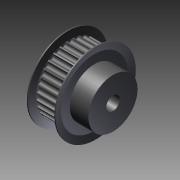
# Autodesk Inventor part: zrr_htd_3m9_6_17023200
Saved by Autodesk Inventor 2011 SP1 (Build 150282100, 282)
## iProperties
Created: 2018-07-07
Part Number: zrr_htd_3m9_6_17023200
Catalog Web Link: www.cadenas.de
Description: zrr_htd_3m9-HTD Pulleys Profile 3M, Timing Belt Width 9 mm
Vendor: MAEDLER
Document SubType Name: Modeling
Designer: psAdmin
Manufacturer: MAEDLER
Mass: 41 g
Surface Area: 52.9577 cm^2
Volume: 10.7438 cm^3
Density: 1 g/cm^3
Category: PARTsolutions
Company: MAEDLER
Title: zrr_htd_3m9_6_17023200
Author: Cadenas PARTsolutions
Comments: HTD Pulleys Profile 3M, Timing Belt Width 9 mm
PSOL_IDENT_0: {$CADENAS_DATA\23d-libs\maedler\antriebselemente\zahnriemenraeder_zahnriemen\zahnriemenraeder\htd-pr
PSOL_IDENT_1: ofil\zrr_htd_3m09.prj},194 {VTYP=3D},{NB=zrr_htd_3m9_6_17023200},{LINA=zrr_htd_3m9_6_17023200},{NN=z
PSOL_IDENT_2: rr_htd_3m9},{DATE=31.01.2018 13:45:46},{GEOMDATE=31.01.2018 13:45:46},{VERSION=},{LINEID=340},{LINES
PSOL_IDENT_3: UBID=-1},{WBVAR=BX}  {NB=zrr_htd_3m9_6_17023200},{LINA=zrr_htd_3m9_6_17023200},{KT=DUMMY},{ARTNR=170
PSOL_IDENT_4: 23200},{PDF=PDF Katalogseite},{AUSF=32-3M-09-1F},{MAT=Aluminium},{ZTL=3.000},{ZRB=9.000},{Z=32.000},
PSOL_IDENT_5: {AUS=1F},{ZS=29.800},{BS=36.000},{DO=30.560},{ND=22.000},{B=12.800},{L=20.600},{I=0.000},{VB=6.000},
PSOL_IDENT_6: {FB=13.500},{BX=6},{GEW=41.000},{ZT=1.200},{ZB=1.800},{T=1.000},{BB=1.000}
NN: zrr_htd_3m9
NT: HTD-Zahnriemenräder Profil 3M, Zahnriemenbreite 9mm
NB: zrr_htd_3m9_6_17023200
NBSYN: zrr_htd_3m9_$BX._$ARTNR.
LINA: zrr_htd_3m9_6_17023200
ARTNR: 17023200
PDF: PDF Katalogseite
AUSF: 32-3M-09-1F
MAT: Aluminium
ZTL: 3.000
ZRB: 9.000
Z: 32.000
AUS: 1F
ZS: 29.800
BS: 36.000
DO: 30.560
ND: 22.000
B: 12.800
L: 20.600
I: 0.000
VB: 6.000
FB: 13.500
BX: 6
GEW: 41.000
ZT: 1.200
ZB: 1.800
T: 1.000
BB: 1.000
SUPPLIER: MAEDLER
ARTICLENO: zrr_htd_3m9_6_17023200
BOMINFO: zrr_htd_3m9_6_17023200
CREATOR: CADENAS GmbH
Autodesk Inventor part; units mm, degrees
ref_plane "YZ Plane" through (0, 0, 0) normal (1, 0, 0) x (0, 1, 0)
ref_plane "XZ Plane" through (0, 0, 0) normal (0, 1, 0) x (-1, 0, 0)
ref_plane "XY Plane" through (0, 0, 0) normal (0, 0, 1) x (1, 0, 0)
sketch "Sketch_3" plane through (0, 0, 0) normal (0, 0, 1) x (1, 0, 0)
  line L0 (500, 0) -> (-500, 0)
  line L1 (0, 0) -> (0, 18)
  line L2 (0, 18) -> (0.4534, 18)
  line L3 (0.4534, 18) -> (1, 14.9)
  line L4 (1, 14.9) -> (11.8, 14.9)
  line L5 (11.8, 14.9) -> (12.3466, 18)
  line L6 (12.3466, 18) -> (12.8, 18)
  line L7 (12.8, 18) -> (12.2534, 14.9)
  line L8 (12.2534, 14.9) -> (12.2534, 11)
  line L9 (12.2534, 11) -> (20.6, 11)
  line L10 (20.6, 11) -> (20.6, 0)
  line L11 (20.6, 0) -> (0, 0)
  constraints: 24 end point
revolve "Revolution1" add sketch "Sketch_3" angle 360 about axis through (500, 0, 0) along (1, 0, 0)
sketch "Sketch_4" plane through (1, 0, 0) normal (1, 0, 0) x (0, 0, -1)
  circle A0 centre (0, 0) radius 206
  arc A1 (-14.8517, -1.199) -> (-14.8283, -1.4605) centre (0, 0) ccw
  arc A2 (-14.8283, -1.4605) -> (-14.8002, -1.7214) centre (0, 0) ccw
  arc A3 (-14.3324, -4.0734) -> (-14.8002, -1.7214) centre (-14.6137, -2.9068) ccw
  arc A4 (-14.3324, -4.0734) -> (-14.2584, -4.3252) centre (0, 0) ccw
  arc A5 (-14.2584, -4.3252) -> (-14.18, -4.5757) centre (0, 0) ccw
  arc A6 (-13.2623, -6.7912) -> (-14.18, -4.5757) centre (-13.7658, -5.702) ccw
  arc A7 (-13.2623, -6.7912) -> (-13.1406, -7.0238) centre (0, 0) ccw
  arc A8 (-13.1406, -7.0238) -> (-13.0149, -7.2542) centre (0, 0) ccw
  arc A9 (-11.6826, -9.2481) -> (-13.0149, -7.2542) centre (-12.3889, -8.278) ccw
  arc A10 (-11.6826, -9.2481) -> (-11.5179, -9.4525) centre (0, 0) ccw
  arc A11 (-11.5179, -9.4525) -> (-11.3496, -9.6539) centre (0, 0) ccw
  arc A12 (-9.6539, -11.3496) -> (-11.3496, -9.6539) centre (-10.5359, -10.5359) ccw
  arc A13 (-9.6539, -11.3496) -> (-9.4525, -11.5179) centre (0, 0) ccw
  arc A14 (-9.4525, -11.5179) -> (-9.2481, -11.6826) centre (0, 0) ccw
  arc A15 (-7.2542, -13.0149) -> (-9.2481, -11.6826) centre (-8.278, -12.3889) ccw
  arc A16 (-7.2542, -13.0149) -> (-7.0238, -13.1406) centre (0, 0) ccw
  arc A17 (-7.0238, -13.1406) -> (-6.7912, -13.2623) centre (0, 0) ccw
  arc A18 (-4.5757, -14.18) -> (-6.7912, -13.2623) centre (-5.702, -13.7658) ccw
  arc A19 (-4.5757, -14.18) -> (-4.3252, -14.2584) centre (0, 0) ccw
  arc A20 (-4.3252, -14.2584) -> (-4.0734, -14.3324) centre (0, 0) ccw
  arc A21 (-1.7214, -14.8002) -> (-4.0734, -14.3324) centre (-2.9068, -14.6137) ccw
  arc A22 (-1.7214, -14.8002) -> (-1.4605, -14.8283) centre (0, 0) ccw
  arc A23 (-1.4605, -14.8283) -> (-1.199, -14.8517) centre (0, 0) ccw
  arc A24 (1.199, -14.8517) -> (-1.199, -14.8517) centre (0, -14.9) ccw
  arc A25 (1.199, -14.8517) -> (1.4605, -14.8283) centre (0, 0) ccw
  arc A26 (1.4605, -14.8283) -> (1.7214, -14.8002) centre (0, 0) ccw
  arc A27 (4.0734, -14.3324) -> (1.7214, -14.8002) centre (2.9068, -14.6137) ccw
  arc A28 (4.0734, -14.3324) -> (4.3252, -14.2584) centre (0, 0) ccw
  arc A29 (4.3252, -14.2584) -> (4.5757, -14.18) centre (0, 0) ccw
  arc A30 (6.7912, -13.2623) -> (4.5757, -14.18) centre (5.702, -13.7658) ccw
  arc A31 (6.7912, -13.2623) -> (7.0238, -13.1406) centre (0, 0) ccw
  arc A32 (7.0238, -13.1406) -> (7.2542, -13.0149) centre (0, 0) ccw
  arc A33 (9.2481, -11.6826) -> (7.2542, -13.0149) centre (8.278, -12.3889) ccw
  arc A34 (9.2481, -11.6826) -> (9.4525, -11.5179) centre (0, 0) ccw
  arc A35 (9.4525, -11.5179) -> (9.6539, -11.3496) centre (0, 0) ccw
  arc A36 (11.3496, -9.6539) -> (9.6539, -11.3496) centre (10.5359, -10.5359) ccw
  arc A37 (11.3496, -9.6539) -> (11.5179, -9.4525) centre (0, 0) ccw
  arc A38 (11.5179, -9.4525) -> (11.6826, -9.2481) centre (0, 0) ccw
  arc A39 (13.0149, -7.2542) -> (11.6826, -9.2481) centre (12.3889, -8.278) ccw
  arc A40 (13.0149, -7.2542) -> (13.1406, -7.0238) centre (0, 0) ccw
  arc A41 (13.1406, -7.0238) -> (13.2623, -6.7912) centre (0, 0) ccw
  arc A42 (14.18, -4.5757) -> (13.2623, -6.7912) centre (13.7658, -5.702) ccw
  arc A43 (14.18, -4.5757) -> (14.2584, -4.3252) centre (0, 0) ccw
  arc A44 (14.2584, -4.3252) -> (14.3324, -4.0734) centre (0, 0) ccw
  arc A45 (14.8002, -1.7214) -> (14.3324, -4.0734) centre (14.6137, -2.9068) ccw
  arc A46 (14.8002, -1.7214) -> (14.8283, -1.4605) centre (0, 0) ccw
  arc A47 (14.8283, -1.4605) -> (14.8517, -1.199) centre (0, 0) ccw
  arc A48 (14.8517, 1.199) -> (14.8517, -1.199) centre (14.9, 0) ccw
  arc A49 (14.8517, 1.199) -> (14.8283, 1.4605) centre (0, 0) ccw
  arc A50 (14.8283, 1.4605) -> (14.8002, 1.7214) centre (0, 0) ccw
  arc A51 (14.3324, 4.0734) -> (14.8002, 1.7214) centre (14.6137, 2.9068) ccw
  arc A52 (14.3324, 4.0734) -> (14.2584, 4.3252) centre (0, 0) ccw
  arc A53 (14.2584, 4.3252) -> (14.18, 4.5757) centre (0, 0) ccw
  arc A54 (13.2623, 6.7912) -> (14.18, 4.5757) centre (13.7658, 5.702) ccw
  arc A55 (13.2623, 6.7912) -> (13.1406, 7.0238) centre (0, 0) ccw
  arc A56 (13.1406, 7.0238) -> (13.0149, 7.2542) centre (0, 0) ccw
  arc A57 (11.6826, 9.2481) -> (13.0149, 7.2542) centre (12.3889, 8.278) ccw
  arc A58 (11.6826, 9.2481) -> (11.5179, 9.4525) centre (0, 0) ccw
  arc A59 (11.5179, 9.4525) -> (11.3496, 9.6539) centre (0, 0) ccw
  arc A60 (9.6539, 11.3496) -> (11.3496, 9.6539) centre (10.5359, 10.5359) ccw
  arc A61 (9.6539, 11.3496) -> (9.4525, 11.5179) centre (0, 0) ccw
  arc A62 (9.4525, 11.5179) -> (9.2481, 11.6826) centre (0, 0) ccw
  arc A63 (7.2542, 13.0149) -> (9.2481, 11.6826) centre (8.278, 12.3889) ccw
  arc A64 (7.2542, 13.0149) -> (7.0238, 13.1406) centre (0, 0) ccw
  arc A65 (7.0238, 13.1406) -> (6.7912, 13.2623) centre (0, 0) ccw
  arc A66 (4.5757, 14.18) -> (6.7912, 13.2623) centre (5.702, 13.7658) ccw
  arc A67 (4.5757, 14.18) -> (4.3252, 14.2584) centre (0, 0) ccw
  arc A68 (4.3252, 14.2584) -> (4.0734, 14.3324) centre (0, 0) ccw
  arc A69 (1.7214, 14.8002) -> (4.0734, 14.3324) centre (2.9068, 14.6137) ccw
  arc A70 (1.7214, 14.8002) -> (1.4605, 14.8283) centre (0, 0) ccw
  arc A71 (1.4605, 14.8283) -> (1.199, 14.8517) centre (0, 0) ccw
  arc A72 (-1.199, 14.8517) -> (1.199, 14.8517) centre (0, 14.9) ccw
  arc A73 (-1.199, 14.8517) -> (-1.4605, 14.8283) centre (0, 0) ccw
  arc A74 (-1.4605, 14.8283) -> (-1.7214, 14.8002) centre (0, 0) ccw
  arc A75 (-4.0734, 14.3324) -> (-1.7214, 14.8002) centre (-2.9068, 14.6137) ccw
  arc A76 (-4.0734, 14.3324) -> (-4.3252, 14.2584) centre (0, 0) ccw
  arc A77 (-4.3252, 14.2584) -> (-4.5757, 14.18) centre (0, 0) ccw
  arc A78 (-6.7912, 13.2623) -> (-4.5757, 14.18) centre (-5.702, 13.7658) ccw
  arc A79 (-6.7912, 13.2623) -> (-7.0238, 13.1406) centre (0, 0) ccw
  arc A80 (-7.0238, 13.1406) -> (-7.2542, 13.0149) centre (0, 0) ccw
  arc A81 (-9.2481, 11.6826) -> (-7.2542, 13.0149) centre (-8.278, 12.3889) ccw
  arc A82 (-9.2481, 11.6826) -> (-9.4525, 11.5179) centre (0, 0) ccw
  arc A83 (-9.4525, 11.5179) -> (-9.6539, 11.3496) centre (0, 0) ccw
  arc A84 (-11.3496, 9.6539) -> (-9.6539, 11.3496) centre (-10.5359, 10.5359) ccw
  arc A85 (-11.3496, 9.6539) -> (-11.5179, 9.4525) centre (0, 0) ccw
  arc A86 (-11.5179, 9.4525) -> (-11.6826, 9.2481) centre (0, 0) ccw
  arc A87 (-13.0149, 7.2542) -> (-11.6826, 9.2481) centre (-12.3889, 8.278) ccw
  arc A88 (-13.0149, 7.2542) -> (-13.1406, 7.0238) centre (0, 0) ccw
  arc A89 (-13.1406, 7.0238) -> (-13.2623, 6.7912) centre (0, 0) ccw
  arc A90 (-14.18, 4.5757) -> (-13.2623, 6.7912) centre (-13.7658, 5.702) ccw
  arc A91 (-14.18, 4.5757) -> (-14.2584, 4.3252) centre (0, 0) ccw
  arc A92 (-14.2584, 4.3252) -> (-14.3324, 4.0734) centre (0, 0) ccw
  arc A93 (-14.8002, 1.7214) -> (-14.3324, 4.0734) centre (-14.6137, 2.9068) ccw
  arc A94 (-14.8002, 1.7214) -> (-14.8283, 1.4605) centre (0, 0) ccw
  arc A95 (-14.8283, 1.4605) -> (-14.8517, 1.199) centre (0, 0) ccw
  arc A96 (-14.8517, -1.199) -> (-14.8517, 1.199) centre (-14.9, 0) ccw
  constraints: 192 point on circle, 97 centre point
extrude "Extrusion1" cut sketch "Sketch_4" along normal blind 10.8
sketch "Sketch_9_ALT_Drilling_1" plane through (0, 0, 0) normal (1, 0, 0) x (0, 1, 0)
  circle A0 centre (0, 0) radius 3
  constraints: 1 centre point
extrude "Extrusion2" cut sketch "Sketch_9_ALT_Drilling_1" along normal blind 20.6
body "Solid1"
